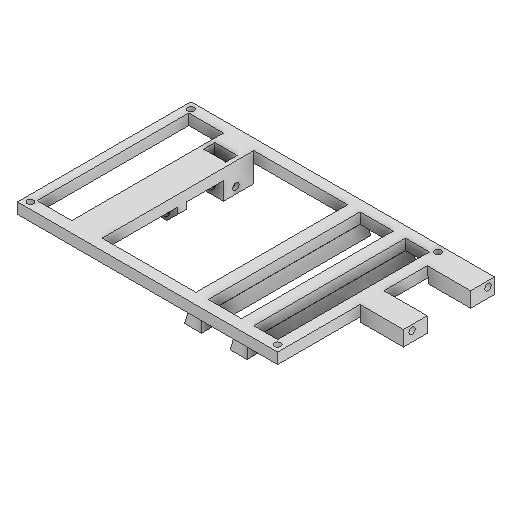
# Autodesk Inventor part: Rail_carriage_v2
Saved by Autodesk Inventor 2023 (Build 270158000, 158)
## iProperties
Created: 2022-01-10
Part Number: Rail_carriage_v2
Material: Generic
Document SubType Name: Modeling
Designer: CDT
Density: 1 g/cm^3
Appearance: Default
Author: CDT
Autodesk Inventor part; units mm, degrees
ref_plane "YZ Plane" through (0, 0, 0) normal (1, 0, 0) x (0, 1, 0)
ref_plane "XZ Plane" through (0, 0, 0) normal (0, 1, 0) x (-1, 0, 0)
ref_plane "XY Plane" through (0, 0, 0) normal (0, 0, 1) x (1, 0, 0)
sketch "Sketch1" plane through (0, 0, 0) normal (0, 1, 0) x (-1, 0, 0)
  line L0 (-26.3037, 95.0681) -> (-146.3037, 95.0681)
  line L1 (-146.3037, 95.0681) -> (-146.3037, 15.0681)
  line L2 (-146.3037, 15.0681) -> (-26.3037, 15.0681)
  line L3 (-26.3037, 15.0681) -> (-26.3037, 95.0681)
  line L4 (-30.3037, 90.0681) -> (-141.3037, 90.0681)
  line L5 (-141.3037, 90.0681) -> (-141.3037, 20.0681)
  line L6 (-141.3037, 20.0681) -> (-30.3037, 20.0681)
  line L7 (-30.3037, 20.0681) -> (-30.3037, 90.0681)
  point P0 (0, 0)
  dimension "d2" = 80
  dimension "d3" = 5
  dimension "d4" = 5
  dimension "d6" = 4
  dimension "d9" = 120
  dimension "d10" = 5
  constraints: 16 end point, 4 parallel, 2 horizontal, 2 perpendicular
  measures "d2" distance between parallel lines of L2 L0
  measures "d3" distance between parallel lines of L0 L4
  measures "d4" distance between parallel lines of L2 L6
  measures "d6" distance between parallel lines of L3 L7
  measures "d9" distance between parallel lines of L1 L3
  measures "d10" distance between parallel lines of L1 L5
extrude "Extrusion1" add sketch "Sketch1" along normal blind 5
sketch "Sketch2" plane through (0, 5, 0) normal (0, 1, 0) x (1, 0, 0)
  line L0 (130.3037, -90.0681) -> (124.6037, -90.0681)
  line L1 (124.6037, -90.0681) -> (124.6037, -20.0681)
  line L2 (124.6037, -20.0681) -> (130.3037, -20.0681)
  line L3 (130.3037, -20.0681) -> (130.3037, -90.0681)
  line L4 (30.3037, -20.0681) -> (141.3037, -20.0681) projected
  line L5 (146.3037, -95.0681) -> (146.3037, -15.0681) projected
  line L6 (141.3037, -90.0681) -> (30.3037, -90.0681) projected
  line L7 (109.3037, -90.0681) -> (103.6037, -90.0681)
  line L8 (103.6037, -90.0681) -> (103.6037, -20.0681)
  line L9 (103.6037, -20.0681) -> (109.3037, -20.0681)
  line L10 (109.3037, -20.0681) -> (109.3037, -90.0681)
  line L11 (26.3037, -15.0681) -> (26.3037, -95.0681) projected
  point P0 (0, 0)
  point P1 (109.3037, -90.0681)
  point P2 (103.6037, -20.0681)
  point P3 (103.6037, -90.0681)
  dimension "d11" = 0
  dimension "d12" = 16
  dimension "d13" = 0
  dimension "d14" = 5.7
  dimension "d16" = 5.7
  dimension "d17" = 0
  dimension "d18" = 0
  dimension "d65" = 37
  constraints: 16 end point, 4 parallel, 2 horizontal, 2 perpendicular
  measures "d11" distance between parallel lines of L4 L2
  measures "d12" distance between parallel lines of L5 L3
  measures "d13" distance between parallel lines of L6 L0
  measures "d14" distance between parallel lines of L1 L3
  measures "d16" distance between parallel lines of L8 L10
  measures "d17" distance between parallel lines of L6 L7
  measures "d18" distance between parallel lines of L4 L9
  measures "d65" distance between parallel lines of L5 L10
extrude "Extrusion2" add sketch "Sketch2" against normal up to surface (5 mm away) contours L0 L1 L2 L3 | L6 L8 L4 L10
sketch "Sketch3" plane through (0, 0, 0) normal (0, -1, 0) x (1, 0, 0)
  line L0 (103.4537, 93.0681) -> (109.1537, 93.0681)
  line L1 (109.1537, 93.0681) -> (109.1537, 17.0681)
  line L2 (109.1537, 17.0681) -> (103.4537, 17.0681)
  line L3 (103.4537, 17.0681) -> (103.4537, 93.0681)
  line L4 (26.3037, 95.0681) -> (146.3037, 95.0681) projected
  line L5 (146.3037, 15.0681) -> (26.3037, 15.0681) projected
  line L6 (26.3037, 15.0681) -> (26.3037, 95.0681) projected
  line L7 (124.4537, 93.0681) -> (130.1537, 93.0681)
  line L8 (130.1537, 93.0681) -> (130.1537, 17.0681)
  line L9 (130.1537, 17.0681) -> (124.4537, 17.0681)
  line L10 (124.4537, 17.0681) -> (124.4537, 93.0681)
  line L11 (146.3037, 95.0681) -> (146.3037, 15.0681) projected
  line L12 (109.3037, 20.0681) -> (109.3037, 90.0681) projected
  line L13 (130.3037, 20.0681) -> (130.3037, 90.0681) projected
  point P0 (0, 0)
  dimension "d21" = 2
  dimension "d22" = 2
  dimension "d23" = 5.7
  dimension "d25" = 5.7
  dimension "d26" = 2
  dimension "d27" = 2
  dimension "d66" = 0.15
  dimension "d67" = 0.15
  constraints: 16 end point, 4 parallel, 2 horizontal, 2 perpendicular
  measures "d21" distance between parallel lines of L4 L0
  measures "d22" distance between parallel lines of L5 L2
  measures "d23" distance between parallel lines of L1 L3
  measures "d25" distance between parallel lines of L8 L10
  measures "d26" distance between parallel lines of L4 L7
  measures "d27" distance between parallel lines of L5 L9
  measures "d66" distance between parallel lines of L12 L1
  measures "d67" distance between parallel lines of L13 L8
extrude "Extrusion3" add sketch "Sketch3" along normal blind 6 draft 9.8 contours L0 L1 L2 L3 | L7 L8 L9 L10
sketch "Sketch4" plane through (0, 5, 0) normal (0, 1, 0) x (1, 0, 0)
  line L0 (46.3037, -15.0681) -> (60.3037, -15.0681)
  line L1 (60.3037, -15.0681) -> (60.3037, -95.0681)
  line L2 (60.3037, -95.0681) -> (46.3037, -95.0681)
  line L3 (46.3037, -95.0681) -> (46.3037, -15.0681)
  line L4 (26.3037, -15.0681) -> (26.3037, -95.0681) projected
  line L5 (146.3037, -15.0681) -> (26.3037, -15.0681) projected
  line L6 (26.3037, -95.0681) -> (146.3037, -95.0681) projected
  point P0 (0, 0)
  dimension "d31" = 20
  dimension "d32" = 14
  dimension "d33" = 0
  dimension "d34" = 0
  constraints: 8 end point, 2 parallel, 1 horizontal, 1 perpendicular
  measures "d31" distance between parallel lines of L4 L3
  measures "d32" distance between parallel lines of L1 L3
  measures "d33" distance between parallel lines of L5 L0
  measures "d34" distance between parallel lines of L6 L2
extrude "Extrusion4" add sketch "Sketch4" against normal up to surface (5 mm away) contours L0 L1 L2 L3
sketch "Sketch5" plane through (0, 0, 0) normal (0, -1, 0) x (1, 0, 0)
  line L0 (46.3037, 34.0681) -> (60.3037, 34.0681)
  line L1 (60.3037, 34.0681) -> (60.3037, 20.0681)
  line L2 (60.3037, 20.0681) -> (46.3037, 20.0681)
  line L3 (46.3037, 20.0681) -> (46.3037, 34.0681)
  line L4 (46.3037, 90.0681) -> (46.3037, 20.0681) projected
  line L5 (60.3037, 20.0681) -> (60.3037, 90.0681) projected
  line L6 (46.3037, 90.0681) -> (30.3037, 90.0681) projected
  line L7 (30.3037, 20.0681) -> (46.3037, 20.0681) projected
  line L8 (46.3037, 51.0681) -> (60.3037, 51.0681)
  line L9 (60.3037, 51.0681) -> (60.3037, 55.0681)
  line L10 (60.3037, 55.0681) -> (46.3037, 55.0681)
  line L11 (46.3037, 55.0681) -> (46.3037, 51.0681)
  line L12 (26.3037, 95.0681) -> (146.3037, 95.0681) projected
  point P0 (0, 0)
  point P1 (60.3037, 55.0681)
  point P2 (46.3037, 51.0681)
  dimension "d37" = 0
  dimension "d38" = 0
  dimension "d43" = 14
  dimension "d44" = 0
  dimension "d191" = 40
  dimension "d192" = 0
  dimension "d193" = 0
  dimension "d194" = 4
  constraints: 16 end point, 4 parallel, 2 horizontal, 2 perpendicular
  measures "d37" distance between parallel lines of L4 L3
  measures "d38" distance between parallel lines of L5 L1
  measures "d43" distance between parallel lines of L2 L0
  measures "d44" distance between parallel lines of L7 L2
  measures "d191" distance between parallel lines of L12 L10
  measures "d192" distance between parallel lines of L4 L11
  measures "d193" distance between parallel lines of L5 L9
  measures "d194" distance between parallel lines of L10 L8
extrude "Extrusion5" add sketch "Sketch5" along normal blind 8.25 contours L0 L1 L2 L3 | L4 L10 L5 L8
sketch "Sketch6" plane through (60.3037, 0, 20.0681) normal (0, 0, -1) x (-1, 0, 0)
  circle A0 centre (7, -3.7) radius 3.25
  line L0 (14, -8.25) -> (0, -8.25) projected
  line L1 (14, 0) -> (14, -8.25) projected
  line L2 (-86, 0) -> (34, 0) projected
  point P0 (60.3037, 0)
  dimension "d45" = 6.5
  dimension "d47" = 7
  dimension "d190" = 3.7
  constraints: 1 centre point
  measures "d45" diameter of A0
  measures "d47" distance from line of L1 A0.centre
  measures "d190" distance from line of L2 A0.centre
extrude "Extrusion6" cut sketch "Sketch6" against normal through all
sketch "Sketch7" plane through (0, -8.25, 0) normal (0, -1, 0) x (1, 0, 0)
  line L0 (48.1537, 25.8681) -> (58.4537, 25.8681)
  line L1 (58.4537, 25.8681) -> (58.4537, 31.0681)
  line L2 (58.4537, 31.0681) -> (48.1537, 31.0681)
  line L3 (48.1537, 31.0681) -> (48.1537, 25.8681)
  line L4 (46.3037, 34.0681) -> (46.3037, 20.0681) projected
  line L5 (46.3037, 20.0681) -> (60.3037, 20.0681) projected
  line L6 (60.3037, 20.0681) -> (60.3037, 34.0681) projected
  line L7 (60.3037, 34.0681) -> (46.3037, 34.0681) projected
  point P0 (0, 0)
  dimension "d50" = 10.3
  dimension "d51" = 5.2
  dimension "d52" = 1.85
  dimension "d56" = 1.85
  dimension "d195" = 3
  constraints: 8 end point, 2 parallel, 1 horizontal, 1 perpendicular
  measures "d50" distance of L2.end L1.end
  measures "d51" distance of L1.end L0.end
  measures "d52" distance between parallel lines of L4 L3
  measures "d56" distance between parallel lines of L6 L1
  measures "d195" distance between parallel lines of L7 L2
extrude "Extrusion7" cut sketch "Sketch7" against normal up to surface (13.25 mm away) contours L3 L2 L1 L0
sketch "Sketch19" plane through (0, 5, 0) normal (0, 1, 0) x (1, 0, 0)
  circle A0 centre (29.3037, -18.0681) radius 1.5
  circle A1 centre (143.3037, -18.0681) radius 1.5
  circle A2 centre (29.3037, -92.0681) radius 1.5
  circle A3 centre (143.3037, -92.0681) radius 1.5
  line L0 (26.3037, -15.0681) -> (26.3037, -95.0681) projected
  line L1 (146.3037, -15.0681) -> (26.3037, -15.0681) projected
  line L2 (146.3037, -95.0681) -> (146.3037, -15.0681) projected
  line L3 (26.3037, -95.0681) -> (146.3037, -95.0681) projected
  point P0 (0, 0)
  dimension "d135" = 3
  dimension "d136" = 3
  dimension "d137" = 3
  dimension "d138" = 3
  dimension "d139" = 3
  dimension "d140" = 3
  dimension "d141" = 3
  dimension "d142" = 3
  dimension "d143" = 3
  dimension "d144" = 3
  dimension "d145" = 3
  dimension "d146" = 3
  constraints: 4 centre point
  measures "d135" diameter of A0
  measures "d136" diameter of A1
  measures "d137" diameter of A2
  measures "d138" diameter of A3
  measures "d139" distance from line of L0 A0.centre
  measures "d140" distance from line of L1 A0.centre
  measures "d141" distance from line of L1 A1.centre
  measures "d142" distance from line of L2 A1.centre
  measures "d143" distance from line of L3 A3.centre
  measures "d144" distance from line of L2 A3.centre
  measures "d145" distance from line of L0 A2.centre
  measures "d146" distance from line of L3 A2.centre
extrude "Extrusion19" cut sketch "Sketch19" against normal blind 10 contours A0 | A1 | A2 | A3
sketch "Sketch22" plane through (0, 5, 0) normal (0, 1, 0) x (1, 0, 0)
  line L0 (146.3037, -95.0681) -> (146.3037, -15.0681) projected
  line L1 (146.3037, -15.0681) -> (166.3037, -15.0681)
  line L2 (166.3037, -15.0681) -> (166.3037, -57.0681)
  line L3 (166.3037, -57.0681) -> (146.3037, -57.0681)
  line L4 (146.3037, -57.0681) -> (146.3037, -15.0681)
  line L5 (166.3037, -46.0681) -> (146.3037, -46.0681)
  line L6 (146.3037, -46.0681) -> (146.3037, -26.0681)
  line L7 (146.3037, -26.0681) -> (166.3037, -26.0681)
  line L8 (166.3037, -26.0681) -> (166.3037, -46.0681)
  point P0 (0, 0)
  dimension "d158" = 20
  dimension "d159" = 42
  dimension "d166" = 20
  dimension "d167" = 11
  dimension "d168" = 11
  dimension "d169" = 0
  dimension "d170" = 0
  constraints: 16 end point, 4 parallel, 2 horizontal, 2 perpendicular
  measures "d158" distance of L2.end L3.end
  measures "d159" distance of L1.end L2.end
  measures "d166" distance between parallel lines of L7 L5
  measures "d167" distance between parallel lines of L1 L7
  measures "d168" distance between parallel lines of L3 L5
  measures "d169" distance between parallel lines of L2 L8
  measures "d170" distance between parallel lines of L0 L6
extrude "Extrusion22" add sketch "Sketch22" against normal blind 4 contours L0 L5 L2 L3 | L0 L1 L2 L7
sketch "Sketch25" plane through (0, 1, 0) normal (0, -1, 0) x (1, 0, 0)
  line L0 (166.3037, 46.0681) -> (166.3037, 57.0681) projected
  line L1 (166.3037, 57.0681) -> (146.7037, 57.0681)
  line L2 (146.7037, 57.0681) -> (146.7037, 46.0681)
  line L3 (146.7037, 46.0681) -> (166.3037, 46.0681)
  line L4 (166.3037, 46.0681) -> (166.3037, 57.0681)
  line L5 (166.3037, 26.0681) -> (146.3037, 26.0681) projected
  line L6 (166.3037, 26.0681) -> (146.7037, 26.0681)
  line L7 (146.7037, 26.0681) -> (146.7037, 15.0681)
  line L8 (146.7037, 15.0681) -> (166.3037, 15.0681)
  line L9 (166.3037, 15.0681) -> (166.3037, 26.0681)
  point P0 (0, 0)
  point P1 (146.7037, 26.0681)
  dimension "d176" = 19.6
  dimension "d177" = 11
  dimension "d178" = 19.6
  dimension "d179" = 11
  constraints: 16 end point, 4 parallel, 2 horizontal, 2 perpendicular
  measures "d176" distance of L3.end L2.end
  measures "d177" distance of L2.end L1.end
  measures "d178" distance of L8.end L7.end
  measures "d179" distance of L7.end L6.end
extrude "Extrusion25" add sketch "Sketch25" along normal blind 3
sketch "Sketch26" plane through (166.3037, 5, 26.0681) normal (1, 0, 0) x (0, 0, -1)
  circle A0 centre (8, -2.5) radius 1.5
  circle A1 centre (-27, -2.5) radius 1.5
  line L0 (11, 0) -> (11, -7) projected
  line L1 (-31, 0) -> (-20, 0) projected
  line L2 (0, 0) -> (11, 0) projected
  point P0 (26.0681, -5)
  dimension "d182" = 3
  dimension "d183" = 3
  dimension "d184" = 3
  dimension "d185" = 35
  dimension "d186" = 2.5
  dimension "d187" = 2.5
  constraints: 2 centre point
  measures "d182" diameter of A0
  measures "d183" diameter of A1
  measures "d184" distance from line of L0 A0.centre
  measures "d185" distance of A0.centre A1.centre
  measures "d186" distance from line of L1 A1.centre
  measures "d187" distance from line of L2 A0.centre
extrude "Extrusion26" cut sketch "Sketch26" against normal blind 12
sketch "Sketch27" plane through (60.3037, 5, 90.0681) normal (1, 0, 0) x (0, 0, -1)
  circle A0 centre (61.7, -10.25) radius 1.5
  line L0 (64.2, -13.25) -> (64.2, 0) projected
  line L1 (70, -13.25) -> (56, -13.25) projected
  point P0 (90.0681, -5)
  dimension "d196" = 3
  dimension "d197" = 2.5
  dimension "d198" = 3
  constraints: 1 centre point
  measures "d196" diameter of A0
  measures "d197" distance from line of L0 A0.centre
  measures "d198" distance from line of L1 A0.centre
extrude "Extrusion27" cut sketch "Sketch27" against normal blind 4
sketch "Sketch28" plane through (0, -8.25, 0) normal (0, -1, 0) x (1, 0, 0)
  line L0 (46.3037, 20.0681) -> (46.3037, 90.0681) projected
  line L1 (60.3037, 34.0681) -> (60.3037, 51.0681) projected
  line L2 (46.3037, 55.0681) -> (60.3037, 55.0681)
  line L3 (60.3037, 55.0681) -> (60.3037, 51.0681)
  line L4 (60.3037, 51.0681) -> (46.3037, 51.0681)
  line L5 (46.3037, 51.0681) -> (46.3037, 55.0681)
  point P0 (0, 0)
  constraints: 8 end point, 2 parallel, 1 horizontal, 1 midpoint, 1 perpendicular
extrude "Extrusion28" cut sketch "Sketch28" against normal blind 0.3
chamfer "Chamfer1" distance 5 angle 45 2 edges at (46.3037, -7.95, 53.0681) (60.3037, -7.95, 53.0681)
equation "\"d3\" = d4"
equation "\"d4\" = d10"
equation "\"d25\" = d23"
equation "\"d26\" = d21"
equation "\"d27\" = d22"
equation "\"d66\" = d67"
equation "\"d176\" = d178"
equation "\"d186\" = d187"
body "Solid1"
